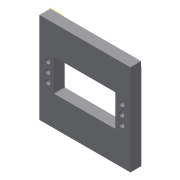
# Autodesk Inventor part: SeroHolderMount1
Saved by Autodesk Inventor 2018 (Build 220112000, 112)
## iProperties
Created: 2018-10-17
Part Number: SeroHolderMount1
Material: Generic
Document SubType Name: Modeling
Designer: Vulnic
Density: 1 g/cm^3
Appearance: Default
Author: Vulnic
Autodesk Inventor part; units mm, degrees
ref_plane "YZ Plane" through (0, 0, 0) normal (1, 0, 0) x (0, 1, 0)
ref_plane "XZ Plane" through (0, 0, 0) normal (0, 1, 0) x (-1, 0, 0)
ref_plane "XY Plane" through (0, 0, 0) normal (0, 0, 1) x (1, 0, 0)
ref_plane "Work Plane1" through (67.4704, 11.9331, 5.1843) normal (0, 0, 1) x (1, 0.0008, 0)
sketch "Sketch1" plane through (67.4704, 11.9331, 5.1843) normal (0, 0, 1) x (1, 0.0008, 0)
  line L0 (0.75, -8.6866) -> (3.5, -8.6866) projected
  arc A0 (0.75, -8.6866) -> (-1.25, -10.6866) centre (0.75, -10.6866) ccw projected
  line L1 (-1.25, -10.6866) -> (-1.25, -18.9366) projected
  arc A1 (-1.25, -18.9366) -> (0.75, -20.9366) centre (0.75, -18.9366) ccw projected
  line L2 (0.75, -20.9366) -> (3.5, -20.9366) projected
  arc A2 (3, -20.4366) -> (3.5, -20.9366) centre (3.5, -20.4366) ccw projected
  line L3 (3, -9.1866) -> (3, -20.4366) projected
  arc A3 (3.5, -8.6866) -> (3, -9.1866) centre (3.5, -9.1866) ccw projected
  circle A4 centre (0.625, -18.3116) radius 1 projected
  circle A5 centre (0.625, -14.8116) radius 1 projected
  circle A6 centre (0.625, -11.3116) radius 1 projected
  line L4 (26.25, -20.9366) -> (29, -20.9366) projected
  arc A7 (29, -20.9366) -> (31, -18.9366) centre (29, -18.9366) ccw projected
  line L5 (31, -10.6866) -> (31, -18.9366) projected
  arc A8 (31, -10.6866) -> (29, -8.6866) centre (29, -10.6866) ccw projected
  line L6 (26.25, -8.6866) -> (29, -8.6866) projected
  arc A9 (26.75, -9.1866) -> (26.25, -8.6866) centre (26.25, -9.1866) ccw projected
  line L7 (26.75, -9.1866) -> (26.75, -20.4366) projected
  arc A10 (26.25, -20.9366) -> (26.75, -20.4366) centre (26.25, -20.4366) ccw projected
  circle A11 centre (29.125, -18.3116) radius 1 projected
  circle A12 centre (29.125, -14.8116) radius 1 projected
  circle A13 centre (29.125, -11.3116) radius 1 projected
  line L8 (32.5, -32.5) -> (-2.5, -32.5) projected
  line L9 (-2.5, -32.5) -> (-2.5, 2.5) projected
  line L10 (-2.5, 2.5) -> (32.5, 2.5) projected
  line L11 (32.5, 2.5) -> (32.5, -32.5) projected
  line L12 (22.05, -20.9366) -> (3.5, -20.9366) projected
  arc A14 (3, -20.4366) -> (3.5, -20.9366) centre (3.5, -20.4366) ccw projected
  line L13 (3, -9.1866) -> (3, -20.4366) projected
  arc A15 (3.5, -8.6866) -> (3, -9.1866) centre (3.5, -9.1866) ccw projected
  line L14 (22.05, -8.6866) -> (3.5, -8.6866) projected
  line L15 (22.05, -8.6866) -> (22.05, -14.2116) projected
  line L16 (19.0411, -14.2116) -> (22.05, -14.2116) projected
  arc A16 (19.0411, -14.2116) -> (16.255, -11.9616) centre (16.255, -14.8116) ccw projected
  line L17 (15.3815, -11.9616) -> (16.255, -11.9616) projected
  arc A17 (15.3815, -11.9616) -> (15.3815, -17.6616) centre (10.13, -14.8116) ccw projected
  line L18 (16.255, -17.6616) -> (15.3815, -17.6616) projected
  arc A18 (16.255, -17.6616) -> (19.0411, -15.4116) centre (16.255, -14.8116) ccw projected
  line L19 (19.0411, -15.4116) -> (22.05, -15.4116) projected
  line L20 (22.05, -15.4116) -> (22.05, -20.9366) projected
  line L21 (26.75, -9.1866) -> (26.75, -20.4366) projected
  arc A19 (26.25, -20.9366) -> (26.75, -20.4366) centre (26.25, -20.4366) ccw projected
  line L22 (26.25, -20.9366) -> (22.05, -20.9366) projected
  line L23 (22.05, -15.4116) -> (22.05, -20.9366) projected
  line L24 (22.05, -15.4116) -> (19.0411, -15.4116) projected
  arc A20 (19.0411, -15.4116) -> (19.0411, -14.2116) centre (16.255, -14.8116) ccw projected
  line L25 (22.05, -14.2116) -> (19.0411, -14.2116) projected
  line L26 (22.05, -8.6866) -> (22.05, -14.2116) projected
  line L27 (26.25, -8.6866) -> (22.05, -8.6866) projected
  arc A21 (26.75, -9.1866) -> (26.25, -8.6866) centre (26.25, -9.1866) ccw projected
  point P0 (-67.4803, -11.8769)
extrude "Extrusion1" add sketch "Sketch1" along normal blind 4.15 contours L0 A3 L3 A2 L2 A1 L1 A0 | L6 A8 L5 A7 L4 A10 L7 A9 | L8 L9 L10 L11
body "Solid1"
